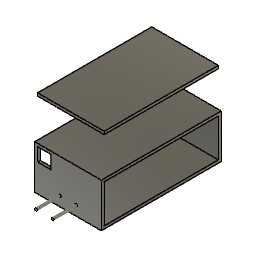
Robot frame v4 (Autodesk Fusion 360 design; units mm, degrees)
Autodesk Fusion 360 part; units mm, degrees
sketch "Sketch1" plane through (0, 0, 0) normal (0, 1, 0) x (1, 0, 0) in component "Frame"
  line L0 (0, 0) -> (-70, 0)
  line L1 (-70, 0) -> (-70, -89)
  line L2 (-70, -89) -> (0, -89)
  line L3 (0, -89) -> (0, 0)
  dimension "d1" = 70
  dimension "d2" = 89
  constraint horizontal L0
  constraint vertical L1
  constraint horizontal L2
  constraint vertical L3
  constraint coincident L0.start L3.end
  measures "d1" distance of L0.start L0.end
  measures "d2" distance of L0.start L2.end
extrude "Extrude1" add sketch "Sketch1" along normal blind 120 makes body 1 in component "Frame"
sketch "Sketch2" plane through (0, 0, 0) normal (0, -1, 0) x (1, 0, 0) in component "Frame"
  line L0 (0, 0) -> (0, 89)
  line L1 (0, 89) -> (-70, 89)
  line L2 (-70, 89) -> (-70, 0)
  line L3 (-70, 0) -> (0, 0)
  line L4 (0, 0) -> (-70, 0)
  line L5 (-70, 0) -> (-70, 46)
  line L6 (-70, 46) -> (0, 46)
  line L7 (0, 46) -> (0, 0)
  dimension "d5" = 70
  dimension "d6" = 46
  constraint horizontal L4
  constraint vertical L5
  constraint horizontal L6
  constraint vertical L7
  constraint coincident L0.start L3.end
  measures "d5" distance of L0.start L2.end
  measures "d6" distance of L0.start L6.end
extrude "Extrude2" add sketch "Sketch2" along normal blind 3 contours L0 L2 L3 L4 L5 L6 L7 bodies 1 in component "Frame"
sketch "Sketch3" plane through (0, 120, 0) normal (0, 1, 0) x (-1, 0, 0) in component "Frame"
  line L0 (0, 89) -> (0, 0)
  line L1 (0, 0) -> (70, 0)
  line L2 (70, 0) -> (70, 89)
  line L3 (70, 89) -> (0, 89)
  line L4 (0, 0) -> (70, 0)
  line L5 (70, 0) -> (70, 46)
  line L6 (70, 46) -> (0, 46)
  line L7 (0, 46) -> (0, 0)
  dimension "d9" = 70
  dimension "d10" = 46
  constraint horizontal L4
  constraint vertical L5
  constraint horizontal L6
  constraint vertical L7
  constraint coincident L0.end L1.start
  measures "d9" distance of L0.end L1.end
  measures "d10" distance of L0.end L6.end
extrude "Extrude3" add sketch "Sketch3" along normal blind 3 contours L0 L1 L2 L4 L5 L6 L7 bodies 1 in component "Frame"
sketch "Sketch4" plane through (0, 120, 0) normal (0, 1, 0) x (-1, 0, 0) in component "Frame"
  line L0 (0, 46) -> (70, 46)
  line L1 (70, 46) -> (70, 89)
  line L2 (70, 89) -> (0, 89)
  line L3 (0, 89) -> (0, 46)
  line L4 (0, 46) -> (67, 46)
  line L5 (67, 46) -> (67, 86)
  line L6 (67, 86) -> (0, 86)
  line L7 (0, 86) -> (0, 46)
  dimension "d13" = 67
  dimension "d14" = 40
  constraint horizontal L4
  constraint vertical L5
  constraint horizontal L6
  constraint vertical L7
  constraint coincident L0.start L3.end
  measures "d13" distance of L0.start L4.end
  measures "d14" distance of L0.start L6.end
extrude "Extrude4" cut sketch "Sketch4" against normal up to surface (120 mm away) contours L0 L3 L4 L5 L6 L7 bodies 1 in component "Frame"
sketch "Sketch5" plane through (0, 0, 0) normal (1, 0, 0) x (0, 1, 0) in component "Frame"
  line L0 (123, 46) -> (-3, 46)
  line L1 (-3, 46) -> (-3, 0)
  line L2 (-3, 0) -> (123, 0)
  line L3 (123, 0) -> (123, 46)
  line L4 (120, 3) -> (0, 3)
  line L5 (0, 3) -> (0, 43)
  line L6 (0, 43) -> (120, 43)
  line L7 (120, 43) -> (120, 3)
  dimension "d17" = 120
  constraint horizontal L4
  constraint vertical L5
  constraint horizontal L6
  constraint vertical L7
  measures "d17" distance of L4.start L4.end
extrude "Extrude5" cut sketch "Sketch5" against normal blind 67 contours L4 L5 L6 L7 bodies 1 in component "Frame"
sketch "Sketch6" plane through (-67, 0, 0) normal (1, 0, 0) x (0, 1, 0) in component "Frame"
  line L0 (120, 43) -> (0, 43)
  line L1 (0, 43) -> (0, 3)
  line L2 (0, 3) -> (120, 3)
  line L3 (120, 3) -> (120, 43)
  line L4 (0, 43) -> (40, 43)
  line L5 (40, 43) -> (40, 3)
  line L6 (40, 3) -> (0, 3)
  line L7 (0, 3) -> (0, 43)
  dimension "d20" = 40
  dimension "d21" = 40
  constraint horizontal L4
  constraint vertical L5
  constraint horizontal L6
  constraint vertical L7
  constraint coincident L0.end L1.start
  measures "d20" distance of L0.end L4.end
  measures "d21" distance of L0.end L1.end
extrude "Extrude6" cut sketch "Sketch6" against normal blind 3 contours L0 L1 L2 L4 L5 L6 L7 bodies 1 in component "Frame"
sketch "Sketch7" plane through (-67, 0, 0) normal (1, 0, 0) x (0, 1, 0) in component "Frame"
  line L0 (40, 43) -> (40, 3)
  line L1 (40, 3) -> (120, 3)
  line L2 (120, 3) -> (120, 43)
  line L3 (120, 43) -> (40, 43)
  line L4 (120, 3) -> (80, 3)
  line L5 (80, 3) -> (80, 43)
  line L6 (80, 43) -> (120, 43)
  line L7 (120, 43) -> (120, 3)
  dimension "d24" = 40
  dimension "d25" = 40
  constraint horizontal L4
  constraint vertical L5
  constraint horizontal L6
  constraint vertical L7
  constraint coincident L1.end L2.start
  measures "d24" distance of L1.end L4.end
  measures "d25" distance of L1.end L2.end
extrude "Extrude7" cut sketch "Sketch7" against normal blind 3 contours L1 L2 L3 L4 L5 L6 L7 bodies 1 in component "Frame"
sketch "Sketch8" plane through (-67, 0, 0) normal (1, 0, 0) x (0, 1, 0) in component "Frame"
  line L0 (0, 86) -> (0, 46)
  line L1 (0, 46) -> (120, 46)
  line L2 (120, 46) -> (120, 86)
  line L3 (120, 86) -> (0, 86)
  line L4 (0, 86) -> (40, 86)
  line L5 (40, 86) -> (40, 46)
  line L6 (40, 46) -> (0, 46)
  line L7 (0, 46) -> (0, 86)
  dimension "d28" = 40
  dimension "d29" = 40
  constraint horizontal L4
  constraint vertical L5
  constraint horizontal L6
  constraint vertical L7
  constraint coincident L0.start L3.end
  measures "d28" distance of L0.start L4.end
  measures "d29" distance of L0.start L0.end
extrude "Extrude8" cut sketch "Sketch8" against normal blind 3 contours L0 L1 L3 L4 L5 L6 L7 bodies 1 in component "Frame"
sketch "Sketch9" plane through (-67, 0, 0) normal (1, 0, 0) x (0, 1, 0) in component "Frame"
  line L0 (40, 86) -> (40, 46)
  line L1 (40, 46) -> (120, 46)
  line L2 (120, 46) -> (120, 86)
  line L3 (120, 86) -> (40, 86)
  line L4 (120, 46) -> (80, 46)
  line L5 (80, 46) -> (80, 86)
  line L6 (80, 86) -> (120, 86)
  line L7 (120, 86) -> (120, 46)
  dimension "d32" = 40
  dimension "d33" = 40
  constraint horizontal L4
  constraint vertical L5
  constraint horizontal L6
  constraint vertical L7
  constraint coincident L1.end L2.start
  measures "d32" distance of L1.end L4.end
  measures "d33" distance of L1.end L2.end
extrude "Extrude9" cut sketch "Sketch9" against normal blind 3 contours L1 L2 L3 L4 L5 L6 L7 bodies 1 in component "Frame"
sketch "Sketch10" plane through (0, -3, 0) normal (0, -1, 0) x (1, 0, 0) in component "Frame"
  line L0 (0, 46) -> (-70, 46)
  line L1 (-70, 46) -> (-70, 0)
  line L2 (-70, 0) -> (0, 0)
  line L3 (0, 0) -> (0, 46)
  line L4 (0, 0) -> (-26.25, 0) construction
  line L5 (-26.25, 0) -> (-26.25, 10) construction
  line L6 (-26.25, 10) -> (-43.75, 10) construction
  line L7 (-43.75, 10) -> (-43.75, 0) construction
  line L8 (-43.75, 0) -> (-70, 0) construction
  circle A0 centre (-43.75, 10) radius 1.45
  circle A1 centre (-26.25, 10) radius 1.45
  dimension "d36" = 26.25
  dimension "d37" = 10
  dimension "d38" = 17.5
  dimension "d39" = 2.9
  dimension "d40" = 2.9
  constraint coincident L2.end L3.start
  constraint coincident L2 L4.end
  constraint perpendicular L4 L5
  constraint perpendicular L1 L6
  constraint coincident L2 L7.end
  constraint perpendicular L2 L7
  constraint coincident L1.end L2.start
  constraint coincident L6.end L7.start
  constraint coincident L5.end L6.start
  measures "d36" distance of L2.end L4.end
  measures "d37" distance of L4.end L5.end
  measures "d38" distance of L5.end L6.end
  measures "d39" diameter of A0
  measures "d40" diameter of A1
extrude "Extrude10" add sketch "Sketch10" along normal blind 25 contours A0 | A1 bodies 1 in component "Frame"
sketch "Sketch11" plane through (0, -3, 0) normal (0, -1, 0) x (1, 0, 0) in component "Frame"
  circle A0 centre (-26.25, 10) radius 1.45
  circle A1 centre (-43.75, 10) radius 1.45
  line L0 (0, 46) -> (-70, 46)
  line L1 (-70, 46) -> (-70, 0)
  line L2 (-70, 0) -> (0, 0)
  line L3 (0, 0) -> (0, 46)
  line L4 (-70, 46) -> (-67, 46) construction
  line L5 (-67, 46) -> (-67, 43) construction
  line L6 (-67, 43) -> (-53, 43)
  line L7 (-53, 43) -> (-53, 29)
  line L8 (-53, 29) -> (-67, 29)
  line L9 (-67, 29) -> (-67, 43)
  dimension "d43" = 3
  constraint coincident L0.end L1.start
  constraint coincident L0 L4.end
  constraint perpendicular L1 L4
  constraint perpendicular L0 L5
  constraint horizontal L6
  constraint vertical L7
  constraint horizontal L8
  constraint vertical L9
  measures "d43" distance of L4.end L5.end
extrude "Extrude11" cut sketch "Sketch11" against normal blind 3 contours L6 L7 L8 L9 bodies 1 in component "Frame"
sketch "Sketch12" plane through (0, 123, 0) normal (0, 1, 0) x (-1, 0, 0) in component "Frame"
  line L0 (0, 46) -> (0, 0)
  line L1 (0, 0) -> (70, 0)
  line L2 (70, 0) -> (70, 46)
  line L3 (70, 46) -> (0, 46)
  line L4 (70, 46) -> (67, 46) construction
  line L5 (67, 46) -> (67, 43) construction
  line L6 (67, 43) -> (53, 43)
  line L7 (53, 43) -> (53, 29)
  line L8 (53, 29) -> (67, 29)
  line L9 (67, 29) -> (67, 43)
  dimension "d46" = 3
  dimension "d47" = 14
  dimension "d48" = 14
  constraint coincident L2.end L3.start
  constraint coincident L3 L4.end
  constraint perpendicular L2 L4
  constraint perpendicular L4 L5
  constraint horizontal L6
  constraint vertical L7
  constraint horizontal L8
  constraint vertical L9
  measures "d46" distance of L4.end L5.end
  measures "d47" distance of L5.end L6.end
  measures "d48" distance of L5.end L8.end
extrude "Extrude12" cut sketch "Sketch12" against normal blind 3 contours L6 L7 L8 L9 bodies 1 in component "Frame"
sketch "Sketch13" plane through (0, 123, 0) normal (0, 1, 0) x (-1, 0, 0) in component "Frame"
  line L0 (53, 43) -> (67, 43)
  line L1 (67, 43) -> (67, 29)
  line L2 (67, 29) -> (53, 29)
  line L3 (53, 29) -> (53, 43)
  line L4 (0, 46) -> (0, 0)
  line L5 (0, 0) -> (70, 0)
  line L6 (70, 0) -> (70, 46)
  line L7 (70, 46) -> (0, 46)
  line L8 (70, 0) -> (43.75, 0) construction
  line L9 (43.75, 0) -> (43.75, 10) construction
  line L10 (43.75, 10) -> (26.25, 10) construction
  line L11 (26.25, 10) -> (26.25, 0) construction
  line L12 (0, 0) -> (26.25, 0) construction
  circle A0 centre (26.25, 10) radius 1.45
  circle A1 centre (43.75, 10) radius 1.45
  dimension "d51" = 26.25
  dimension "d52" = 10
  dimension "d53" = 17.5
  dimension "d54" = 2.9
  dimension "d55" = 2.9
  constraint coincident L5.end L6.start
  constraint perpendicular L6 L8
  constraint perpendicular L8 L9
  constraint perpendicular L9 L10
  constraint coincident L5 L11.end
  constraint perpendicular L5 L11
  constraint coincident L4.end L5.start
  constraint coincident L10.end L11.start
  constraint coincident L9.end L10.start
  measures "d51" distance of L5.end L8.end
  measures "d52" distance of L8.end L9.end
  measures "d53" distance of L9.end L10.end
  measures "d54" diameter of A0
  measures "d55" diameter of A1
extrude "Extrude13" add sketch "Sketch13" along normal blind 25 contours A0 | A1 bodies 1 in component "Frame"
sketch "Sketch1 (2)" plane through (0, 0, 0) normal (0, 1, 0) x (1, 0, 0) in component "Frame partial"
  line L0 (0, 0) -> (-70, 0)
  line L1 (-70, 0) -> (-70, -89)
  line L2 (-70, -89) -> (0, -89)
  line L3 (0, -89) -> (0, 0)
  dimension "d1_1" = 70
  dimension "d2_1" = 89
  constraint horizontal L0
  constraint vertical L1
  constraint horizontal L2
  constraint vertical L3
  constraint coincident L0.start L3.end
  measures "d1_1" distance of L0.start L0.end
  measures "d2_1" distance of L0.start L2.end
extrude "Extrude1'" add sketch "Sketch1 (2)" along normal blind 120 separate body makes body 2 in component "Frame partial"
sketch "Sketch2 (2)" plane through (0, 0, 0) normal (0, -1, 0) x (1, 0, 0) in component "Frame partial"
  line L0 (0, 0) -> (0, 89)
  line L1 (0, 89) -> (-70, 89)
  line L2 (-70, 89) -> (-70, 0)
  line L3 (-70, 0) -> (0, 0)
  line L4 (0, 0) -> (-70, 0)
  line L5 (-70, 0) -> (-70, 46)
  line L6 (-70, 46) -> (0, 46)
  line L7 (0, 46) -> (0, 0)
  dimension "d5_1" = 70
  dimension "d6_1" = 46
  constraint horizontal L4
  constraint vertical L5
  constraint horizontal L6
  constraint vertical L7
  constraint coincident L0.start L3.end
  measures "d5_1" distance of L0.start L2.end
  measures "d6_1" distance of L0.start L6.end
extrude "Extrude2'" add sketch "Sketch2 (2)" along normal blind 3 contours L0 L2 L3 L4 L5 L6 L7 bodies 2 in component "Frame partial"
sketch "Sketch3 (2)" plane through (0, 120, 0) normal (0, 1, 0) x (-1, 0, 0) in component "Frame partial"
  line L0 (0, 89) -> (0, 0)
  line L1 (0, 0) -> (70, 0)
  line L2 (70, 0) -> (70, 89)
  line L3 (70, 89) -> (0, 89)
  line L4 (0, 0) -> (70, 0)
  line L5 (70, 0) -> (70, 46)
  line L6 (70, 46) -> (0, 46)
  line L7 (0, 46) -> (0, 0)
  dimension "d9_1" = 70
  dimension "d10_1" = 46
  constraint horizontal L4
  constraint vertical L5
  constraint horizontal L6
  constraint vertical L7
  constraint coincident L0.end L1.start
  measures "d9_1" distance of L0.end L1.end
  measures "d10_1" distance of L0.end L6.end
extrude "Extrude3'" add sketch "Sketch3 (2)" along normal blind 3 contours L0 L1 L2 L4 L5 L6 L7 bodies 2 in component "Frame partial"
sketch "Sketch4 (2)" plane through (0, 120, 0) normal (0, 1, 0) x (-1, 0, 0) in component "Frame partial"
  line L0 (0, 46) -> (70, 46)
  line L1 (70, 46) -> (70, 89)
  line L2 (70, 89) -> (0, 89)
  line L3 (0, 89) -> (0, 46)
  line L4 (0, 46) -> (67, 46)
  line L5 (67, 46) -> (67, 86)
  line L6 (67, 86) -> (0, 86)
  line L7 (0, 86) -> (0, 46)
  dimension "d13_1" = 67
  dimension "d14_1" = 40
  constraint horizontal L4
  constraint vertical L5
  constraint horizontal L6
  constraint vertical L7
  constraint coincident L0.start L3.end
  measures "d13_1" distance of L0.start L4.end
  measures "d14_1" distance of L0.start L6.end
extrude "Extrude4'" cut sketch "Sketch4 (2)" against normal up to surface (120 mm away) contours L0 L3 L4 L5 L6 L7 bodies 2 in component "Frame partial"
sketch "Sketch5 (2)" plane through (0, 0, 0) normal (1, 0, 0) x (0, 1, 0) in component "Frame partial"
  line L0 (123, 46) -> (-3, 46)
  line L1 (-3, 46) -> (-3, 0)
  line L2 (-3, 0) -> (123, 0)
  line L3 (123, 0) -> (123, 46)
  line L4 (120, 3) -> (0, 3)
  line L5 (0, 3) -> (0, 43)
  line L6 (0, 43) -> (120, 43)
  line L7 (120, 43) -> (120, 3)
  dimension "d17_1" = 120
  constraint horizontal L4
  constraint vertical L5
  constraint horizontal L6
  constraint vertical L7
  measures "d17_1" distance of L4.start L4.end
extrude "Extrude5'" cut sketch "Sketch5 (2)" against normal blind 67 contours L4 L5 L6 L7 bodies 2 in component "Frame partial"
sketch "Sketch6 (2)" plane through (-67, 0, 0) normal (1, 0, 0) x (0, 1, 0) in component "Frame partial"
  line L0 (120, 43) -> (0, 43)
  line L1 (0, 43) -> (0, 3)
  line L2 (0, 3) -> (120, 3)
  line L3 (120, 3) -> (120, 43)
  line L4 (0, 43) -> (40, 43)
  line L5 (40, 43) -> (40, 3)
  line L6 (40, 3) -> (0, 3)
  line L7 (0, 3) -> (0, 43)
  dimension "d20_1" = 40
  dimension "d21_1" = 40
  constraint horizontal L4
  constraint vertical L5
  constraint horizontal L6
  constraint vertical L7
  constraint coincident L0.end L1.start
  measures "d20_1" distance of L0.end L4.end
  measures "d21_1" distance of L0.end L1.end
extrude "Extrude6'" cut sketch "Sketch6 (2)" against normal blind 3 contours L0 L1 L2 L4 L5 L6 L7 bodies 2 in component "Frame partial"
sketch "Sketch7 (2)" plane through (-67, 0, 0) normal (1, 0, 0) x (0, 1, 0) in component "Frame partial"
  line L0 (40, 43) -> (40, 3)
  line L1 (40, 3) -> (120, 3)
  line L2 (120, 3) -> (120, 43)
  line L3 (120, 43) -> (40, 43)
  line L4 (120, 3) -> (80, 3)
  line L5 (80, 3) -> (80, 43)
  line L6 (80, 43) -> (120, 43)
  line L7 (120, 43) -> (120, 3)
  dimension "d24_1" = 40
  dimension "d25_1" = 40
  constraint horizontal L4
  constraint vertical L5
  constraint horizontal L6
  constraint vertical L7
  constraint coincident L1.end L2.start
  measures "d24_1" distance of L1.end L4.end
  measures "d25_1" distance of L1.end L2.end
extrude "Extrude7'" cut sketch "Sketch7 (2)" against normal blind 3 contours L1 L2 L3 L4 L5 L6 L7 bodies 2 in component "Frame partial"
sketch "Sketch8 (2)" plane through (-67, 0, 0) normal (1, 0, 0) x (0, 1, 0) in component "Frame partial"
  line L0 (0, 86) -> (0, 46)
  line L1 (0, 46) -> (120, 46)
  line L2 (120, 46) -> (120, 86)
  line L3 (120, 86) -> (0, 86)
  line L4 (0, 86) -> (40, 86)
  line L5 (40, 86) -> (40, 46)
  line L6 (40, 46) -> (0, 46)
  line L7 (0, 46) -> (0, 86)
  dimension "d28_1" = 40
  dimension "d29_1" = 40
  constraint horizontal L4
  constraint vertical L5
  constraint horizontal L6
  constraint vertical L7
  constraint coincident L0.start L3.end
  measures "d28_1" distance of L0.start L4.end
  measures "d29_1" distance of L0.start L0.end
extrude "Extrude8'" cut sketch "Sketch8 (2)" against normal blind 3 contours L0 L1 L3 L4 L5 L6 L7 bodies 2 in component "Frame partial"
sketch "Sketch9 (2)" plane through (-67, 0, 0) normal (1, 0, 0) x (0, 1, 0) in component "Frame partial"
  line L0 (40, 86) -> (40, 46)
  line L1 (40, 46) -> (120, 46)
  line L2 (120, 46) -> (120, 86)
  line L3 (120, 86) -> (40, 86)
  line L4 (120, 46) -> (80, 46)
  line L5 (80, 46) -> (80, 86)
  line L6 (80, 86) -> (120, 86)
  line L7 (120, 86) -> (120, 46)
  dimension "d32_1" = 40
  dimension "d33_1" = 40
  constraint horizontal L4
  constraint vertical L5
  constraint horizontal L6
  constraint vertical L7
  constraint coincident L1.end L2.start
  measures "d32_1" distance of L1.end L4.end
  measures "d33_1" distance of L1.end L2.end
extrude "Extrude9'" cut sketch "Sketch9 (2)" against normal blind 3 contours L1 L2 L3 L4 L5 L6 L7 bodies 2 in component "Frame partial"
sketch "Sketch10 (2)" plane through (0, -3, 0) normal (0, -1, 0) x (1, 0, 0) in component "Frame partial"
  line L0 (0, 46) -> (-70, 46)
  line L1 (-70, 46) -> (-70, 0)
  line L2 (-70, 0) -> (0, 0)
  line L3 (0, 0) -> (0, 46)
  line L4 (0, 0) -> (-26.25, 0) construction
  line L5 (-26.25, 0) -> (-26.25, 10) construction
  line L6 (-26.25, 10) -> (-43.75, 10) construction
  line L7 (-43.75, 10) -> (-43.75, 0) construction
  line L8 (-43.75, 0) -> (-70, 0) construction
  circle A0 centre (-43.75, 10) radius 1.45
  circle A1 centre (-26.25, 10) radius 1.45
  dimension "d36_1" = 26.25
  dimension "d37_1" = 10
  dimension "d38_1" = 17.5
  dimension "d39_1" = 2.9
  dimension "d40_1" = 2.9
  constraint coincident L2.end L3.start
  constraint coincident L2 L4.end
  constraint perpendicular L4 L5
  constraint perpendicular L1 L6
  constraint coincident L2 L7.end
  constraint perpendicular L2 L7
  constraint coincident L1.end L2.start
  constraint coincident L6.end L7.start
  constraint coincident L5.end L6.start
  measures "d36_1" distance of L2.end L4.end
  measures "d37_1" distance of L4.end L5.end
  measures "d38_1" distance of L5.end L6.end
  measures "d39_1" diameter of A0
  measures "d40_1" diameter of A1
extrude "Extrude10'" add sketch "Sketch10 (2)" along normal blind 25 contours A0 | A1 bodies 2 in component "Frame partial"
sketch "Sketch11 (2)" plane through (0, -3, 0) normal (0, -1, 0) x (1, 0, 0) in component "Frame partial"
  circle A0 centre (-26.25, 10) radius 1.45
  circle A1 centre (-43.75, 10) radius 1.45
  line L0 (0, 46) -> (-70, 46)
  line L1 (-70, 46) -> (-70, 0)
  line L2 (-70, 0) -> (0, 0)
  line L3 (0, 0) -> (0, 46)
  line L4 (-70, 46) -> (-67, 46) construction
  line L5 (-67, 46) -> (-67, 43) construction
  line L6 (-67, 43) -> (-53, 43)
  line L7 (-53, 43) -> (-53, 29)
  line L8 (-53, 29) -> (-67, 29)
  line L9 (-67, 29) -> (-67, 43)
  dimension "d43_1" = 3
  constraint coincident L0.end L1.start
  constraint coincident L0 L4.end
  constraint perpendicular L1 L4
  constraint perpendicular L0 L5
  constraint horizontal L6
  constraint vertical L7
  constraint horizontal L8
  constraint vertical L9
  measures "d43_1" distance of L4.end L5.end
extrude "Extrude11'" cut sketch "Sketch11 (2)" against normal blind 3 contours L6 L7 L8 L9 bodies 2 in component "Frame partial"
sketch "Sketch12 (2)" plane through (0, 123, 0) normal (0, 1, 0) x (-1, 0, 0) in component "Frame partial"
  line L0 (0, 46) -> (0, 0)
  line L1 (0, 0) -> (70, 0)
  line L2 (70, 0) -> (70, 46)
  line L3 (70, 46) -> (0, 46)
  line L4 (70, 46) -> (67, 46) construction
  line L5 (67, 46) -> (67, 43) construction
  line L6 (67, 43) -> (53, 43)
  line L7 (53, 43) -> (53, 29)
  line L8 (53, 29) -> (67, 29)
  line L9 (67, 29) -> (67, 43)
  dimension "d46_1" = 3
  dimension "d47_1" = 14
  dimension "d48_1" = 14
  constraint coincident L2.end L3.start
  constraint coincident L3 L4.end
  constraint perpendicular L2 L4
  constraint perpendicular L4 L5
  constraint horizontal L6
  constraint vertical L7
  constraint horizontal L8
  constraint vertical L9
  measures "d46_1" distance of L4.end L5.end
  measures "d47_1" distance of L5.end L6.end
  measures "d48_1" distance of L5.end L8.end
extrude "Extrude12'" cut sketch "Sketch12 (2)" against normal blind 3 contours L6 L7 L8 L9 bodies 2 in component "Frame partial"
sketch "Sketch13 (2)" plane through (0, 123, 0) normal (0, 1, 0) x (-1, 0, 0) in component "Frame partial"
  line L0 (53, 43) -> (67, 43)
  line L1 (67, 43) -> (67, 29)
  line L2 (67, 29) -> (53, 29)
  line L3 (53, 29) -> (53, 43)
  line L4 (0, 46) -> (0, 0)
  line L5 (0, 0) -> (70, 0)
  line L6 (70, 0) -> (70, 46)
  line L7 (70, 46) -> (0, 46)
  line L8 (70, 0) -> (43.75, 0) construction
  line L9 (43.75, 0) -> (43.75, 10) construction
  line L10 (43.75, 10) -> (26.25, 10) construction
  line L11 (26.25, 10) -> (26.25, 0) construction
  line L12 (0, 0) -> (26.25, 0) construction
  circle A0 centre (26.25, 10) radius 1.45
  circle A1 centre (43.75, 10) radius 1.45
  dimension "d51_1" = 26.25
  dimension "d52_1" = 10
  dimension "d53_1" = 17.5
  dimension "d54_1" = 2.9
  dimension "d55_1" = 2.9
  constraint coincident L5.end L6.start
  constraint perpendicular L6 L8
  constraint perpendicular L8 L9
  constraint perpendicular L9 L10
  constraint coincident L5 L11.end
  constraint perpendicular L5 L11
  constraint coincident L4.end L5.start
  constraint coincident L10.end L11.start
  constraint coincident L9.end L10.start
  measures "d51_1" distance of L5.end L8.end
  measures "d52_1" distance of L8.end L9.end
  measures "d53_1" distance of L9.end L10.end
  measures "d54_1" diameter of A0
  measures "d55_1" diameter of A1
extrude "Extrude13'" add sketch "Sketch13 (2)" along normal blind 25 contours A0 | A1 bodies 2 in component "Frame partial"
sketch "Sketch14" plane through (-70, 0, 0) normal (-1, 0, 0) x (0, -1, 0) in component "Frame"
  line L0 (155, 46) -> (112, 46)
  line L1 (112, 46) -> (112, 0)
  line L2 (112, 0) -> (238, 0)
  line L3 (238, 0) -> (238, 46)
  line L4 (238, 46) -> (195, 46)
  line L5 (195, 46) -> (195, 86)
  line L6 (195, 86) -> (235, 86)
  line L7 (235, 86) -> (235, 89)
  line L8 (235, 89) -> (115, 89)
  line L9 (115, 89) -> (115, 86)
  line L10 (115, 86) -> (155, 86)
  line L11 (155, 86) -> (155, 46)
  line L12 (155, 43) -> (155, 3)
  line L13 (155, 3) -> (115, 3)
  line L14 (115, 3) -> (115, 43)
  line L15 (115, 43) -> (155, 43)
  line L16 (195, 3) -> (195, 43)
  line L17 (195, 43) -> (235, 43)
  line L18 (235, 43) -> (235, 3)
  line L19 (235, 3) -> (195, 3)
  line L20 (115, 0) -> (271.3047, 0)
  line L21 (271.3047, 0) -> (271.3047, 99.153)
  line L22 (271.3047, 99.153) -> (115, 99.153)
  line L23 (115, 99.153) -> (115, 0)
  constraint horizontal L20
  constraint vertical L21
  constraint horizontal L22
  constraint vertical L23
  constraint coincident L2 L20.start
extrude "Extrude14" cut sketch "Sketch14" against normal blind 70 contours L0 L2 L3 L4 L5 L6 L7 L8 L9 L10 L11 L12 L13 L15 L20 L23 | L0 L10 L11 L23 | L12 L13 L14 L15 L23 | L3 L4 L5 L6 L7 L8 L20 L21 L22 L23 | L16 L17 L18 L19 sketch seen with x (1, 0, 0) y (0, 1, 0) z (0, 0, 1) at (0, 235, 0) bodies 2 in component "Frame partial"
sketch "Sketch14 (2)" plane through (0, 123, 0) normal (0, 1, 0) x (-1, 0, 0) in component "Frame partial"
  circle A0 centre (43.75, 10) radius 1.45
  circle A1 centre (26.25, 10) radius 1.45
  line L0 (53, 43) -> (67, 43)
  line L1 (67, 43) -> (67, 29)
  line L2 (67, 29) -> (53, 29)
  line L3 (53, 29) -> (53, 43)
  line L4 (0, 46) -> (0, 0)
  line L5 (0, 0) -> (70, 0)
  line L6 (70, 0) -> (70, 46)
  line L7 (70, 46) -> (0, 46)
  line L8 (23, 6) -> (47, 6)
  line L9 (47, 6) -> (47, 14)
  line L10 (47, 14) -> (23, 14)
  line L11 (23, 14) -> (23, 6)
  constraint horizontal L8
  constraint vertical L9
  constraint horizontal L10
  constraint vertical L11
extrude "Extrude15" cut sketch "Sketch14 (2)" against normal blind 3 contours L4 L5 L6 L7 bodies 2 in component "Frame partial"
component "Frame" placed x (1, 0, 0) y (0, 1, 0) z (0, 0, 1) at (0, 0, 0)
component "Frame partial" placed x (1, 0, 0) y (0, 1, 0) z (0, 0, 1) at (0, -235, 0)
